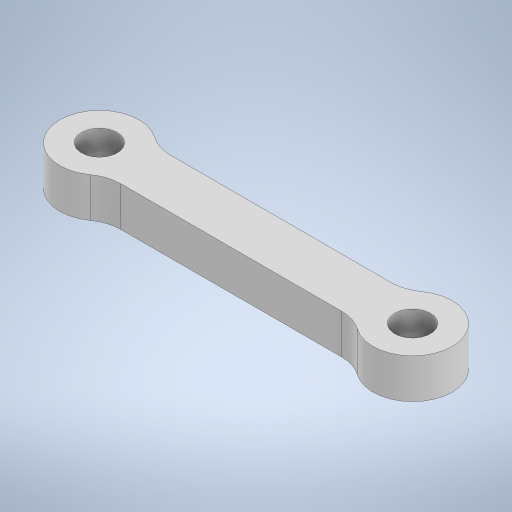
# Autodesk Inventor part: grip link 1
Saved by Autodesk Inventor 2024.1 (Build 281209000, 209)
## iProperties
Created: 2023-12-01
Part Number: grip link 1
Material: Generic
Document SubType Name: Modeling
Designer: vilas
Density: 1 g/cm^3
Appearance: Default
Author: vilas
Autodesk Inventor part; units mm, degrees
ref_plane "YZ Plane" through (0, 0, 0) normal (1, 0, 0) x (0, 1, 0)
ref_plane "XZ Plane" through (0, 0, 0) normal (0, 1, 0) x (-1, 0, 0)
ref_plane "XY Plane" through (0, 0, 0) normal (0, 0, 1) x (1, 0, 0)
sketch "Sketch1" plane through (0, 0, 0) normal (0, 1, 0) x (-1, 0, 0)
  line L0 (-784.4147, 162.8493) -> (-150.5396, 162.8493)
  line L1 (-784.4147, 37.8493) -> (-150.5396, 37.8493)
  line L2 (-467.4771, 37.8493) -> (-467.4771, 162.8493) construction
  line L3 (-467.4771, 100.3493) -> (206.8482, 100.3493) construction
  line L4 (-467.4771, 100.3493) -> (-1186.3819, 100.3493) construction
  circle A0 centre (-72.4771, 100.3493) radius 45
  circle A1 centre (-862.4771, 100.3493) radius 45
  arc A2 (-784.4147, 162.8493) -> (-784.4147, 37.8493) centre (-862.4771, 100.3493) ccw
  arc A3 (-150.5396, 37.8493) -> (-150.5396, 162.8493) centre (-72.4771, 100.3493) ccw
  point P0 (0, 0)
  dimension "d0" = 125
  dimension "d1" = 90
  dimension "d2" = 90
  dimension "d3" = 395
  dimension "d4" = 395
  dimension "d5" = 200
  dimension "d6" = 200
  constraints: 10 end point, 4 centre point, 4 point on circle, 3 midpoint, 2 coincident, 2 horizontal, 2 point on line, 1 vertical
  measures "d0" distance between parallel lines of L1 L0
  measures "d1" diameter of A0
  measures "d2" diameter of A1
  measures "d3" distance from line of L2 A1.centre
  measures "d4" distance from line of A0.centre L2
  measures "d5" diameter of A2
  measures "d6" diameter of A3
extrude "Extrusion1" add sketch "Sketch1" along normal blind 100
fillet "Fillet1" radius 100 4 edges at (784.4147, 50, 37.8493) (150.5396, 50, 37.8493) (150.5396, 50, 162.8493) (784.4147, 50, 162.8493)
scale "Scale1" factors (0.1, 0.1, 0.1) then translate (420.7294, 90, 34.0644) bodies 1
body "Solid1"
